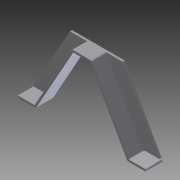
# Autodesk Inventor part: bunny throw base 1
Saved by Autodesk Inventor 2012 (Build 160160000, 160)
## iProperties
Created: 2013-10-11
Part Number: bunny throw base 1
Material: Default
Document SubType Name: Modeling
Designer: Bryce
Density: 1 g/cm^3
Author: Bryce
Autodesk Inventor part; units mm, degrees
ref_plane "YZ Plane" through (0, 0, 0) normal (1, 0, 0) x (0, 1, 0)
ref_plane "XZ Plane" through (0, 0, 0) normal (0, 1, 0) x (-1, 0, 0)
ref_plane "XY Plane" through (0, 0, 0) normal (0, 0, 1) x (1, 0, 0)
sketch "Sketch1" plane through (0, 0, 0) normal (0, 0, 1) x (1, 0, 0)
  line L0 (0, 0) -> (193.675, 0)
  line L1 (84.1375, 101.6) -> (109.5375, 101.6)
  line L2 (84.1375, 101.6) -> (27.3259, 0)
  line L3 (109.5375, 101.6) -> (166.3491, 0)
  line L4 (56.8116, 104.775) -> (0.8877, 4.7625)
  line L5 (136.8634, 104.775) -> (192.7873, 4.7625)
  line L6 (0, 0) -> (0, 3.175)
  line L7 (0, 3.175) -> (25.4636, 3.175)
  line L8 (193.675, 0) -> (193.675, 3.175)
  line L9 (193.675, 3.175) -> (168.2114, 3.175)
  line L10 (168.2114, 3.175) -> (111.3998, 104.775)
  line L11 (111.3998, 104.775) -> (82.2752, 104.775)
  line L12 (82.2752, 104.775) -> (25.4636, 3.175)
  line L13 (56.8116, 104.775) -> (82.2752, 104.775)
  line L14 (111.3998, 104.775) -> (136.8634, 104.775)
  line L15 (0.8877, 4.7625) -> (24.0886, 4.7625)
  line L16 (192.7873, 4.7625) -> (169.5864, 4.7625)
  arc A0 (24.0886, 3.175) -> (24.0886, 4.7625) centre (24.0886, 3.9688) ccw
  arc A1 (169.5864, 4.7625) -> (169.5864, 3.175) centre (169.5864, 3.9688) ccw
  dimension "d0" = 193.675
  dimension "d1" = 25.4
  dimension "d2" = 25.4
  dimension "d3" = 25.4
  dimension "d4" = 3.175
  dimension "d5" = 3.175
  dimension "d6" = 101.6
  dimension "d7" = 1.5875
  dimension "d8" = 1.5875
  dimension "d9" = 1.5875
  constraints: 34 end point, 8 point on line, 4 parallel, 4 perpendicular, 4 point on circle, 4 tangent, 3 collinear, 2 centre point, 2 horizontal alignment, 1 equal length, 1 horizontal, 2 other
  measures "d0" distance of L0.start L0.end
  measures "d1" distance of L1.start L1.end
  measures "d2" distance between parallel lines of L2 L4
  measures "d3" distance between parallel lines of L5 L3
  measures "d4" distance of L0.start L6.end
  measures "d5" distance between parallel lines of L11 L1
  measures "d6" distance between parallel lines of L0 L1
  measures "d7" distance between parallel lines of L7 L15
  measures "d8" distance from line of L10 A1.centre
  measures "d9" distance from line of L12 A0.centre
extrude "Extrusion1" add sketch "Sketch1" along normal blind 25.4 contours L6 L7 L12 L11 L10 L9 L8 L0 L3 L1 L2
extrude "Extrusion2" add sketch "Sketch1" along normal blind 3.175 contours A0 L15 L4 L13 L12 L7 | L9 L10 L14 L5 L16 A1
fillet "Fillet1" radius 1.5875 4 edges at (168.2114, 3.175, 14.2875) (25.4636, 3.175, 14.2875) (84.1375, 101.6, 12.7) (109.5375, 101.6, 12.7)
fillet "Fillet2" radius 3.175 4 edges at (82.2752, 104.775, 14.2875) (111.3998, 104.775, 14.2875) (27.3259, 0, 12.7) (166.3491, 0, 12.7)
equation "\"d5\" = d4"
equation "\"d7\" = 0.5 * d4"
equation "\"d9\" = d8"
body "Solid1"
